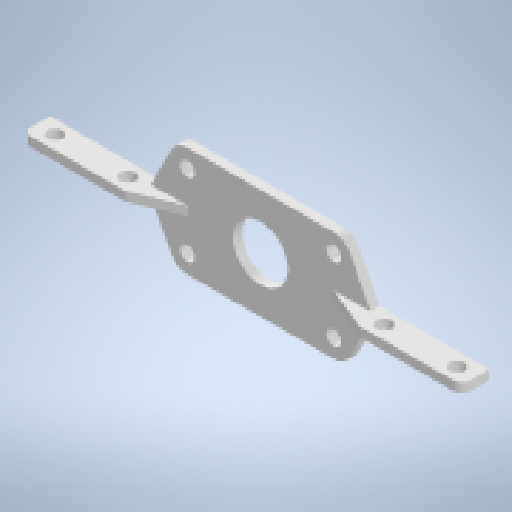
# Autodesk Inventor part: Face Plate
Saved by Autodesk Inventor 2023 (Build 270158000, 158)
## iProperties
Created: 2023-02-27
Part Number: Face Plate
Material: Generic
Document SubType Name: Modeling
Designer: Gabriel - T3 CAD
Density: 1 g/cm^3
Appearance: Default
Author: Gabriel - T3 CAD
Autodesk Inventor part; units mm, degrees
ref_plane "YZ Plane" through (0, 0, 0) normal (1, 0, 0) x (0, 1, 0)
ref_plane "XZ Plane" through (0, 0, 0) normal (0, 1, 0) x (-1, 0, 0)
ref_plane "XY Plane" through (0, 0, 0) normal (0, 0, 1) x (1, 0, 0)
sketch "Sketch1" plane through (0, 0, 0) normal (0, 1, 0) x (-1, 0, 0)
  line L0 (0, 0) -> (152.4, 0)
  line L1 (152.4, 0) -> (152.4, 6.35)
  line L2 (34.925, 9.525) -> (3.175, 9.525)
  line L3 (0, 6.35) -> (0, 0)
  circle A0 centre (6.35, 4.7625) radius 2.5797
  circle A1 centre (31.75, 4.7625) radius 2.5797
  circle A2 centre (120.65, 4.7625) radius 2.5797
  circle A3 centre (146.05, 4.7625) radius 2.5797
  line L4 (38.1, 9.525) -> (114.3, 9.525)
  line L5 (114.3, 6.35) -> (114.3, 4.7625)
  line L6 (38.1, 4.7625) -> (38.1, 6.35)
  arc A4 (38.1, 6.35) -> (34.925, 9.525) centre (34.925, 6.35) ccw
  arc A5 (3.175, 9.525) -> (0, 6.35) centre (3.175, 6.35) ccw
  line L7 (117.475, 9.525) -> (149.225, 9.525)
  arc A6 (117.475, 9.525) -> (114.3, 6.35) centre (117.475, 6.35) ccw
  arc A7 (152.4, 6.35) -> (149.225, 9.525) centre (149.225, 6.35) ccw
  line L8 (114.3, 6.35) -> (114.3, 0)
  line L9 (38.1, 6.35) -> (38.1, 0)
  line L10 (114.3, 4.7625) -> (114.3, 9.525)
  line L11 (117.475, 9.525) -> (114.3, 9.525)
  line L12 (38.1, 6.35) -> (38.1, 9.525)
  line L13 (38.1, 9.525) -> (34.925, 9.525)
  line L14 (38.1, 3.175) -> (114.3, 3.175)
  line L15 (101.6, 3.175) -> (116.2538, 9.2808)
  line L16 (50.8, 3.175) -> (36.1462, 9.2808)
  point P0 (152.4, 9.525)
  point P1 (0, 9.525)
  point P2 (114.3, 3.175)
  dimension "d0" = 152.4
  dimension "d1" = 9.525
  dimension "d2" = 4.7625
  dimension "d3" = 4.7625
  dimension "d4" = 4.7625
  dimension "d5" = 4.7625
  dimension "d6" = 25.4
  dimension "d7" = 25.4
  dimension "d8" = 5.1594
  dimension "d9" = 6.35
  dimension "d10" = 6.35
  dimension "d11" = 4.7625
  dimension "d12" = 6.35
  dimension "d13" = 6.35
  dimension "d14" = 3.175
  dimension "d15" = 3.175
  dimension "d37" = 3.175
  dimension "d100" = 12.7
  constraints: 34 end point, 13 point on line, 12 tangent, 10 point on circle, 8 centre point, 7 perpendicular, 5 equal radius, 3 horizontal, 3 midpoint, 3 parallel, 1 equal length
  measures "d0" distance of point (152.4, 9.525) point (0, 9.525)
  measures "d1" distance of L0.end point (152.4, 9.525)
  measures "d2" distance from line of L0 A0.centre
  measures "d3" distance from line of L0 A1.centre
  measures "d4" distance from line of L0 A2.centre
  measures "d5" distance from line of L0 A3.centre
  measures "d6" distance of A0.centre A1.centre
  measures "d7" distance of A2.centre A3.centre
  measures "d8" diameter of A3
  measures "d9" distance from line of L3 A0.centre
  measures "d10" distance from line of L1 A3.centre
  measures "d11" distance of L6.start L4.start
  measures "d12" distance from line of A1.centre L6
  measures "d13" distance from line of A2.centre L5
  measures "d14" radius of A4
  measures "d15" radius of A6
  measures "d37" distance between parallel lines of L14 L0
  measures "d100" distance of point (114.3, 3.175) L15.start
extrude "Extrusion1" add sketch "Sketch1" along normal mid plane 3.175 contours L3 A5 L2 A4 L6 L9 L0 | L9 L14 L8 L0 | L8 L5 A6 L7 A7 L1 L0 | L9 L6 L12 L16 L14 | L14 L15 L10 L5 L8 | A4 L16 L12 | L10 L15 A6
extrude "Extrusion2" add sketch "Sketch1" along normal mid plane 50.8 contours L9 L14 L8 L0
sketch "Sketch4" plane through (-38.1, 25.4, 0) normal (0, 0, -1) x (-1, 0, 0)
  line L0 (76.2, -50.8) -> (76.2, -26.9875) projected
  line L1 (0, 0) -> (76.2, 0)
  line L2 (76.2, 0) -> (76.2, -50.8)
  line L3 (76.2, -50.8) -> (0, -50.8)
  line L4 (0, -50.8) -> (0, 0)
  circle A0 centre (38.1, -25.4) radius 9.525
  circle A1 centre (12.7, -12.7) radius 2.5797
  circle A2 centre (12.7, -38.1) radius 2.5797
  circle A3 centre (63.5, -12.7) radius 2.5797
  circle A4 centre (63.5, -38.1) radius 2.5797
  circle A5 centre (12.7, -12.7) radius 6.35
  circle A6 centre (12.7, -38.1) radius 6.35
  circle A7 centre (63.5, -12.7) radius 6.35
  circle A8 centre (63.5, -38.1) radius 6.35
  line L5 (12.7, -6.35) -> (63.5, -6.35)
  line L6 (69.85, -11.1925) -> (69.85, -39.6075)
  line L7 (63.5, -44.45) -> (12.7, -44.45)
  line L8 (6.35, -39.6075) -> (6.35, -11.1925)
  line L9 (-38.1, -23.8125) -> (6.35, -23.8125)
  line L10 (6.35, -23.8125) -> (6.35, -26.9875)
  line L11 (6.35, -26.9875) -> (-38.1, -26.9875)
  line L12 (-38.1, -26.9875) -> (-38.1, -23.8125)
  line L13 (69.85, -23.8125) -> (114.3, -23.8125)
  line L14 (114.3, -23.8125) -> (114.3, -26.9875)
  line L15 (114.3, -26.9875) -> (69.85, -26.9875)
  line L16 (69.85, -26.9875) -> (69.85, -23.8125)
  line L17 (-38.1, -26.9875) -> (-38.1, -23.8125) projected
  line L18 (0, -26.9875) -> (-38.1, -26.9875) projected
  line L19 (3.175, -23.8125) -> (6.5632, -11.0684)
  line L20 (3.175, -26.9875) -> (6.5632, -39.7316)
  line L21 (69.6368, -11.0684) -> (73.025, -23.8125)
  line L22 (73.025, -26.9875) -> (69.6368, -39.7316)
  point P0 (-38.1, -25.4)
  point P1 (-38.1, -25.4)
  point P2 (7.0276, -9.8458)
  point P3 (0, -23.8125)
  point P4 (7.0276, -40.9542)
  point P5 (76.2, -23.8125)
  point P6 (69.1724, -9.8458)
  point P7 (69.1724, -40.9542)
  point P8 (0, -23.8125)
  dimension "d71" = 76.2
  dimension "d72" = 50.8
  dimension "d73" = 25.4
  dimension "d74" = 38.1
  dimension "d75" = 19.05
  dimension "d78" = 25.4
  dimension "d81" = 50.8
  dimension "d84" = 12.7
  dimension "d85" = 12.7
  dimension "d86" = 5.1594
  dimension "d87" = 12.7
  dimension "d90" = 25.4
  dimension "d93" = 50.8
  dimension "d96" = 1.5875
  dimension "d97" = 3.175
  dimension "d111" = 3.175
  constraints: 40 end point, 12 point on circle, 9 centre point, 8 parallel, 8 tangent, 6 horizontal, 6 point on line, 4 collinear, 4 equal length, 4 perpendicular, 2 coincident, 2 midpoint, 2 vertical, 12 other
  measures "d71" distance between parallel lines of L0 L4
  measures "d72" distance between parallel lines of L1 L3
  measures "d73" distance from line of L3 point (38.1, -25.4)
  measures "d74" distance from line of L4 point (38.1, -25.4)
  measures "d75" diameter of A0
  measures "d78" distance of A1.centre A2.centre
  measures "d81" distance of A1.centre A3.centre
  measures "d84" distance from line of L1 A1.centre
  measures "d85" distance from line of L4 A1.centre
  measures "d86" diameter of A1
  measures "d87" diameter of A5
  measures "d90" distance of A5.centre A6.centre
  measures "d93" distance of A5.centre A7.centre
  measures "d96" distance from line of A0.centre L11
  measures "d97" distance of L11.end L9.start
  measures "d111" distance of L9.end L19.start
extrude "Extrusion5" cut sketch "Sketch4" against normal blind 3.175 contours L3 L4 L11 L20 A6 L7 A8 L22 L15 L0 | L13 L21 A7 L5 A5 L19 L9 L4 L1 L2 | A0 | A1 | A2 | A3 | A4
equation "\"d2\" = 0.5 * d1"
equation "\"d3\" = d2"
equation "\"d4\" = d2"
equation "\"d5\" = d2"
equation "\"d10\" = d9"
equation "\"d11\" = 0.5 * d1"
equation "\"d37\" = 0.333333 * d1"
body "Solid1"
